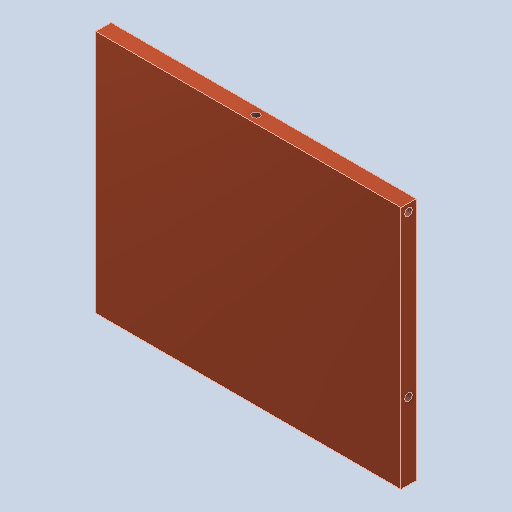
# Autodesk Inventor part: chassis_face_arriere
Saved by Autodesk Inventor 2026.2 (Build 302298010, 298A)
## iProperties
Created: 2026-03-16
Part Number: chassis_face_arriere
Material: Générique
Document SubType Name: Modeling
Designer: genon
Density: 1 g/cm^3
Appearance: Cuivre - Satiné
Author: genon
Autodesk Inventor part; units mm, degrees
ref_plane "YZ Plane" through (0, 0, 0) normal (1, 0, 0) x (0, 1, 0)
ref_plane "XZ Plane" through (0, 0, 0) normal (0, 1, 0) x (-1, 0, 0)
ref_plane "XY Plane" through (0, 0, 0) normal (0, 0, 1) x (1, 0, 0)
sketch "Esquisse1" plane through (0, 0, 0) normal (0, 0, 1) x (1, 0, 0)
  line L0 (0, 0) -> (100, 0)
  line L1 (100, 0) -> (100, 80)
  line L2 (100, 80) -> (0, 80)
  line L3 (0, 80) -> (0, 0)
  dimension "d0" = 100
  dimension "d1" = 80
  constraints: 8 end point, 2 parallel, 1 horizontal, 1 perpendicular
  measures "d0" distance of L2.end L1.end
  measures "d1" distance of L1.end L0.end
extrude "Extrusion1" add sketch "Esquisse1" against normal blind 5
sketch "Esquisse3" plane through (100, 0, 0) normal (1, 0, 0) x (0, 0, -1)
  line L0 (0, 0) -> (0, 80) projected
  line L1 (0, 80) -> (0, 77.5)
  line L2 (0, 77.5) -> (2.5, 77.5)
  line L3 (0, 77.5) -> (2.5, 77.5) construction
  line L4 (0, 0) -> (2.5, 0)
  line L5 (2.5, 0) -> (2.5, 25)
  dimension "d4" = 2.5
  dimension "d5" = 2.5
  dimension "d6" = 0
  dimension "d14" = 25
  constraints: 10 end point, 3 horizontal, 2 coincident, 1 collinear, 1 perpendicular, 1 point on line
  measures "d4" distance of L0.end L1.end
  measures "d5" distance of L1.end L2.end
  measures "d6" distance between parallel lines of L2 L3
  measures "d14" distance of L4.end L5.end
hole "Perçage1" at (100, 77.5, -2.5) at (100, 25, -2.5) direction (-1, 0, 0) diameter 2.459 depth 8.8 tip angle 118 thread size "M3x0.5" class "6H" standard "ISO Metric profile"
sketch "Esquisse4" plane through (0, 0, 0) normal (-1, 0, 0) x (0, 0, 1)
  line L0 (0, 0) -> (-2.5, 0)
  line L1 (0, 0) -> (-5, 0) projected
  line L2 (-2.5, 0) -> (-2.5, 25)
  line L3 (0, 0) -> (0, 80) projected
  line L4 (0, 80) -> (-2.5, 80)
  line L5 (-2.5, 80) -> (-2.5, 77.5)
  dimension "d15" = 2.5
  dimension "d16" = 25
  dimension "d17" = 2.5
  dimension "d18" = 90
  constraints: 8 end point, 2 coincident, 2 perpendicular, 1 horizontal, 1 midpoint
  measures "d15" distance of L0.start L0.end
  measures "d16" distance of L0.end L2.end
  measures "d17" distance of L4.end L5.end
  measures "d18" angle of L5 L4
hole "Perçage2" at (0, 25, -2.5) at (0, 77.5, -2.5) direction (1, 0, 0) diameter 2.459 depth 8.8 tip angle 118 thread size "M3x0.5" class "6H" standard "ISO Metric profile"
sketch "Esquisse5" plane through (0, 80, 0) normal (0, 1, 0) x (1, 0, 0)
  line L0 (100, 0) -> (0, 0) projected
  line L1 (100, 5) -> (0, 5) projected
  line L2 (0, 0) -> (0, 2.5)
  line L3 (0, 0) -> (0, 5) projected
  line L4 (0, 2.5) -> (50, 2.5)
  point P0 (50, 2.5)
  dimension "d41" = 50
  constraints: 4 end point, 1 coincident, 1 midpoint, 1 perpendicular
  measures "d41" distance of L2.end L4.end
hole "Perçage3" at (50, 80, -2.5) direction (0, -1, 0) diameter 2.459 depth 8.8 tip angle 118 thread size "M3x0.5" class "6H" standard "ISO Metric profile"
sketch "Esquisse6" plane through (0, 0, 0) normal (0, -1, 0) x (1, 0, 0)
  line L0 (0, 0) -> (100, 0) projected
  line L1 (0, -5) -> (100, -5) projected
  line L2 (0, 0) -> (0, -2.5)
  line L3 (0, -2.5) -> (50, -2.5)
  point P0 (50, -2.5)
  dimension "d40" = 50
  constraints: 4 end point, 1 coincident, 1 perpendicular, 1 vertical
  measures "d40" distance of L2.end L3.end
hole "Perçage4" at (50, 0, -2.5) direction (0, 1, 0) diameter 2.459 depth 8.8 tip angle 118 thread size "M3x0.5" class "6H" standard "ISO Metric profile"
